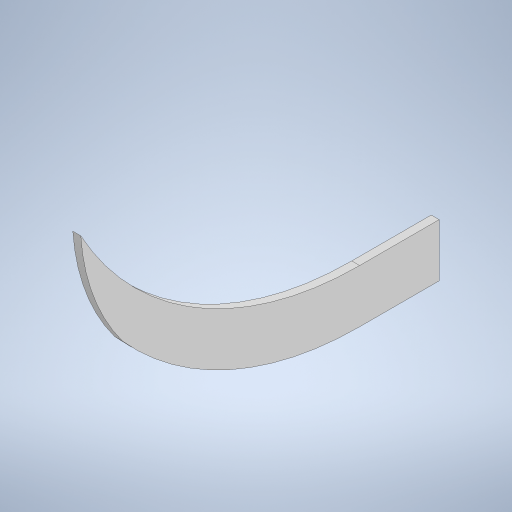
# Autodesk Inventor part: claw
Saved by Autodesk Inventor 2024.1 (Build 281209000, 209)
## iProperties
Created: 2024-02-14
Part Number: claw
Material: 一般
Document SubType Name: Modeling
Designer: hibik
Density: 1 g/cm^3
Appearance: 既定
Author: hibik
Autodesk Inventor part; units mm, degrees
ref_plane "YZ Plane" through (0, 0, 0) normal (1, 0, 0) x (0, 1, 0)
ref_plane "XZ Plane" through (0, 0, 0) normal (0, 1, 0) x (-1, 0, 0)
ref_plane "XY Plane" through (0, 0, 0) normal (0, 0, 1) x (1, 0, 0)
sketch "スケッチ1" plane through (0, 0, 0) normal (1, 0, 0) x (0, 1, 0)
  line L0 (10, 0) -> (0, 0)
  line L1 (0, 0) -> (0, -15)
  line L2 (0, -15) -> (10, -15)
  line L3 (10, -15) -> (10, 0)
  arc A0 (25.2786, 40) -> (10, 0) centre (70, 0) ccw
  arc A1 (20, 44.7214) -> (0, 0) centre (60, 0) ccw
  line L4 (25.2786, 40) -> (20, 44.7214)
  line L5 (70, 0) -> (25.2786, 40) construction
  arc A2 (41.1696, 52.6195) -> (25.2786, 40) centre (70, 0) ccw
  arc A3 (41.1696, 52.6195) -> (20, 44.7214) centre (43.9976, 12.7196) ccw
  dimension "d0" = 10
  dimension "d1" = 15
  dimension "d2" = 60
  dimension "d3" = 60
  dimension "d5" = 40
  dimension "d6" = 20
  dimension "d7" = 40
  constraints: 12 end point, 8 point on circle, 4 centre point, 2 coincident, 2 parallel, 2 tangent, 1 collinear, 1 concentric, 1 horizontal, 1 perpendicular
  measures "d0" distance of L0.start L0.end
  measures "d1" distance of L2.end L0.start
  measures "d2" radius of A0
  measures "d3" radius of A1
  measures "d5" distance from line of L0 L4.start
  measures "d6" distance from line of L4 A2.start
  measures "d7" radius of A3
extrude "押し出し1" add sketch "スケッチ1" along normal blind 1.5
equation "\"d3\" = d2"
